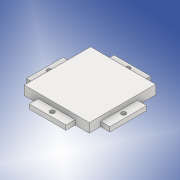
# Autodesk Inventor part: SP002
Saved by Autodesk Inventor 2017 SP1 (Build 210196100, 196)
## iProperties
Created: 2017-08-09
Part Number: SP002
Material: ABS Plastic
Document SubType Name: Modeling
Designer: Zach
Density: 1.06 g/cm^3
Appearance: CR White
Author: Zach
Autodesk Inventor part; units mm, degrees
ref_plane "YZ Plane" through (0, 0, 0) normal (1, 0, 0) x (0, 1, 0)
ref_plane "XZ Plane" through (0, 0, 0) normal (0, 1, 0) x (-1, 0, 0)
ref_plane "XY Plane" through (0, 0, 0) normal (0, 0, 1) x (1, 0, 0)
sketch "Sketch1" plane through (0, 0, 0) normal (0, 0, 1) x (1, 0, 0)
  line L0 (0, 0) -> (71, 0)
  line L1 (71, 0) -> (71, 72.4)
  line L2 (71, 72.4) -> (0, 72.4)
  line L3 (0, 72.4) -> (0, 0)
  dimension "d0" = 71
  dimension "d1" = 72.4
  constraints: 8 end point, 2 parallel, 1 horizontal, 1 perpendicular
  measures "d0" distance of L2.end L1.end
  measures "d1" distance of L0.end L1.end
extrude "Extrusion1" add sketch "Sketch1" along normal blind 10
sketch "Sketch2" plane through (0, 0, 10) normal (0, 0, 1) x (1, 0, 0)
  line L0 (71, 0) -> (71, 72.4) projected
  line L1 (71, 12.4) -> (81, 12.4)
  line L2 (81, 12.4) -> (81, 52.4)
  line L3 (81, 52.4) -> (71, 52.4)
  line L4 (71, 52.4) -> (71, 12.4)
  line L5 (71, 72.4) -> (0, 72.4) projected
  circle A0 centre (76, 32.4) radius 2.5
  line L6 (0, 0) -> (71, 0) projected
  point P0 (81, 32.4)
  point P1 (76, 52.4)
  dimension "d4" = 10
  dimension "d5" = 40
  dimension "d7" = 5
  dimension "d53" = 20
  constraints: 8 end point, 2 midpoint, 2 parallel, 1 centre point, 1 horizontal, 1 horizontal alignment, 1 perpendicular, 1 point on line, 1 vertical alignment
  measures "d4" distance of L3.end L2.end
  measures "d5" distance of L2.end L1.end
  measures "d7" diameter of A0
  measures "d53" distance between parallel lines of L3 L5
extrude "Extrusion2" add sketch "Sketch2" against normal blind 10
sketch "Sketch3" plane through (0, 0, 10) normal (0, 0, 1) x (1, 0, 0)
  line L0 (71, 52.4) -> (81, 52.4) projected
  line L1 (71, 12.4) -> (81, 12.4) projected
  line L2 (81, 52.4) -> (71, 52.4)
  line L3 (71, 52.4) -> (71, 12.4)
  line L4 (71, 12.4) -> (81, 12.4)
  line L5 (81, 12.4) -> (81, 52.4)
  point P0 (0, 0)
  constraints: 8 end point, 2 parallel, 1 horizontal, 1 perpendicular
extrude "Extrusion3" cut sketch "Sketch3" against normal blind 5
sketch "Sketch10" plane through (0, 0, 0) normal (0, 0, -1) x (-1, 0, 0)
  line L0 (0, 72.4) -> (0, 0) projected
  line L1 (0, 12.4) -> (10, 12.4)
  line L2 (10, 12.4) -> (10, 52.4)
  line L3 (10, 52.4) -> (0, 52.4)
  line L4 (0, 52.4) -> (0, 12.4)
  circle A0 centre (5, 32.4) radius 2.5
  point P0 (-81, 12.4)
  point P1 (10, 32.4)
  point P2 (5, 12.4)
  dimension "d40" = 10
  dimension "d41" = 40
  dimension "d42" = 5
  constraints: 8 end point, 2 horizontal alignment, 2 midpoint, 2 parallel, 1 centre point, 1 horizontal, 1 perpendicular, 1 point on line, 1 vertical alignment
  measures "d40" distance of L3.end L2.end
  measures "d41" distance of L2.end L1.end
  measures "d42" diameter of A0
extrude "Extrusion10" add sketch "Sketch10" against normal blind 5
sketch "Sketch11" plane through (0, 0, 0) normal (0, 0, -1) x (-1, 0, 0)
  line L0 (-71, 72.4) -> (0, 72.4) projected
  line L1 (-15.5, 72.4) -> (-55.5, 72.4)
  line L2 (-55.5, 72.4) -> (-55.5, 82.4)
  line L3 (-55.5, 82.4) -> (-15.5, 82.4)
  line L4 (-15.5, 82.4) -> (-15.5, 72.4)
  circle A0 centre (-35.5, 77.4) radius 2.5
  point P0 (0, 0)
  point P1 (-35.5, 82.4)
  point P2 (-35.5, 72.4)
  point P3 (-15.5, 77.4)
  dimension "d46" = 40
  dimension "d47" = 10
  dimension "d48" = 5
  constraints: 8 end point, 3 midpoint, 2 parallel, 2 vertical alignment, 1 centre point, 1 horizontal, 1 horizontal alignment, 1 perpendicular, 1 point on line
  measures "d46" distance of L2.end L3.end
  measures "d47" distance of L1.end L2.end
  measures "d48" diameter of A0
extrude "Extrusion11" add sketch "Sketch11" against normal blind 5
sketch "Sketch12" plane through (0, 0, 0) normal (0, 0, -1) x (-1, 0, 0)
  line L0 (0, 0) -> (-71, 0) projected
  line L1 (-55.5, 0) -> (-15.5, 0)
  line L2 (-15.5, 0) -> (-15.5, -10)
  line L3 (-15.5, -10) -> (-55.5, -10)
  line L4 (-55.5, -10) -> (-55.5, 0)
  circle A0 centre (-35.5, -5) radius 2.5
  point P0 (-55.5, 82.4)
  point P1 (-15.5, 82.4)
  point P2 (-35.5, -10)
  point P3 (-55.5, -5)
  dimension "d54" = 10
  dimension "d55" = 5
  constraints: 8 end point, 3 vertical alignment, 2 midpoint, 2 parallel, 1 centre point, 1 horizontal, 1 horizontal alignment, 1 perpendicular, 1 point on line
  measures "d54" distance of L1.end L2.end
  measures "d55" diameter of A0
extrude "Extrusion12" add sketch "Sketch12" against normal blind 5
body "Solid1"
